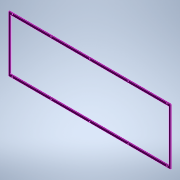
# Autodesk Inventor part: AluminumCasing
Saved by Autodesk Inventor 2021 (Build 250183000, 183)
## iProperties
Created: 2022-02-04
Part Number: AluminumCasing
Material: Generic
Document SubType Name: Modeling
Designer: tlar613
Density: 1 g/cm^3
Appearance: Default
Author: tlar613
Autodesk Inventor part; units mm, degrees
ref_plane "YZ Plane" through (0, 0, 0) normal (1, 0, 0) x (0, 1, 0)
ref_plane "XZ Plane" through (0, 0, 0) normal (0, 1, 0) x (-1, 0, 0)
ref_plane "XY Plane" through (0, 0, 0) normal (0, 0, 1) x (1, 0, 0)
sketch "Sketch1" plane through (0, 0, 0) normal (0, 0, 1) x (1, 0, 0)
  line L0 (-438.2, 150) -> (490, 150)
  line L1 (490, 150) -> (490, -150)
  line L2 (490, -150) -> (-438.2, -150)
  line L3 (-438.2, -150) -> (-438.2, 150)
  line L4 (-448.2, 165) -> (500, 165)
  line L5 (500, 165) -> (500, -165)
  line L6 (500, -165) -> (-448.2, -165)
  line L7 (-448.2, -165) -> (-448.2, 165)
  line L8 (0, 231) -> (0, -231) projected
  line L9 (-637.84, 0) -> (689.64, 0) projected
  line L10 (-448.2, 159) -> (500, 159) construction
  line L11 (500, -159) -> (-448.2, -159) construction
  circle A0 centre (-426.1, -159) radius 3
  circle A1 centre (-200.1, -159) radius 3
  circle A2 centre (25.9, -159) radius 3
  circle A3 centre (251.9, -159) radius 3
  circle A4 centre (477.9, -159) radius 3
  circle A5 centre (-426.1, 159) radius 3
  circle A6 centre (-200.1, 159) radius 3
  circle A7 centre (25.9, 159) radius 3
  circle A8 centre (251.9, 159) radius 3
  circle A9 centre (477.9, 159) radius 3
  point P0 (0, 0)
  dimension "d0" = 928.2
  dimension "d1" = 300
  dimension "d2" = 948.2
  dimension "d3" = 330
  dimension "d6" = 490
  dimension "d7" = 500
  dimension "d8" = 6
  dimension "d9" = 6
  dimension "d10" = 6
  dimension "d11" = 22.1
  dimension "d12" = 226
  dimension "d13" = 226
  dimension "d14" = 226
  dimension "d15" = 226
  dimension "d16" = 22.1
  dimension "d17" = 226
  dimension "d18" = 226
  dimension "d19" = 226
  dimension "d20" = 226
  constraints: 20 end point, 12 point on line, 10 centre point, 9 equal radius, 4 parallel, 4 perpendicular, 2 horizontal, 2 midpoint, 2 other
  measures "d0" distance of L0.start L0.end
  measures "d1" distance of L0.end L1.end
  measures "d2" distance of L4.start L4.end
  measures "d3" distance of L4.end L5.end
  measures "d6" distance between parallel lines of L8 L1
  measures "d7" distance between parallel lines of L8 L5
  measures "d8" distance between parallel lines of L4 L10
  measures "d9" distance between parallel lines of L6 L11
  measures "d10" diameter of A0
  measures "d11" distance from line of L7 A0.centre
  measures "d12" distance of A1.centre A0.centre
  measures "d13" distance of A2.centre A1.centre
  measures "d14" distance of A3.centre A2.centre
  measures "d15" distance of A4.centre A3.centre
  measures "d16" distance from line of L7 A5.centre
  measures "d17" distance of A6.centre A5.centre
  measures "d18" distance of A7.centre A6.centre
  measures "d19" distance of A8.centre A7.centre
  measures "d20" distance of A9.centre A8.centre
extrude "Extrusion1" add sketch "Sketch1" along normal blind 5 contours L3 L9 L7 L4 L8 L0 | L8 L4 L5 L9 L1 L0 | L3 L2 L8 L6 L7 L9 | L9 L5 L6 L8 L2 L1
body "Solid1"
